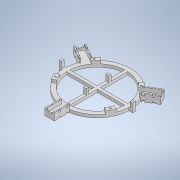
# Autodesk Inventor part: bottom2
Saved by Autodesk Inventor 2020.2 (Build 242310000, 310)
## iProperties
Created: 2020-03-22
Part Number: bottom2
Material: Generic
Document SubType Name: Modeling
Designer: Tarsoly
Density: 1 g/cm^3
Appearance: Default
Author: Tarsoly
Autodesk Inventor part; units mm, degrees
ref_plane "YZ Plane" through (0, 0, 0) normal (1, 0, 0) x (0, 1, 0)
sketch "Sketch1" plane through (0, 0, 0) normal (0, 1, 0) x (-1, 0, 0)
  circle A0 centre (0, 0) radius 57
  circle A1 centre (0, 0) radius 50
  line L0 (0, -84.8) -> (0, 109.8) construction
  line L1 (105.0197, 0) -> (-105.0197, 0) construction
  line L2 (8, 82) -> (-8, 82)
  line L3 (-8, 82) -> (-8, 50)
  line L4 (-8, 50) -> (8, 50)
  line L5 (8, 50) -> (8, 82)
  line L6 (0, 82) -> (0, 50) construction
  circle A2 centre (0, 0) radius 53.5 construction
  circle A3 centre (40.4629, -35) radius 1.5
  circle A4 centre (-40.4629, -35) radius 1.5
  circle A5 centre (-47.2996, 25) radius 1.5
  circle A6 centre (47.2996, 25) radius 1.5
  line L7 (-75.0141, -34.0718) -> (-67.0141, -47.9282)
  line L8 (-39.3013, -31.9282) -> (-47.3013, -18.0718)
  line L9 (-67.0141, -47.9282) -> (-39.3013, -31.9282)
  line L10 (-71.0141, -41) -> (-43.3013, -25) construction
  line L11 (-47.3013, -18.0718) -> (-75.0141, -34.0718)
  line L12 (67.0141, -47.9282) -> (75.0141, -34.0718)
  line L13 (47.3013, -18.0718) -> (39.3013, -31.9282)
  line L14 (75.0141, -34.0718) -> (47.3013, -18.0718)
  line L15 (71.0141, -41) -> (43.3013, -25) construction
  line L16 (39.3013, -31.9282) -> (67.0141, -47.9282)
  point P0 (-8, 56.4358)
  point P1 (8, 56.4358)
  point P2 (-44.8748, -35.1461)
  point P3 (-52.8748, -21.2897)
  point P4 (52.8748, -21.2897)
  point P5 (44.8748, -35.1461)
  dimension "d0" = 114
  dimension "d1" = 100
  dimension "d10" = 16
  dimension "d61" = 107
  dimension "d62" = 3
  dimension "d63" = 3
  dimension "d64" = 3
  dimension "d65" = 3
  dimension "d66" = 35
  dimension "d67" = 35
  dimension "d68" = 25
  dimension "d69" = 25
  dimension "d71" = 32
  dimension "d92" = 360
  constraints: 30 end point, 7 centre point, 4 point on circle, 3 coincident, 2 midpoint, 2 parallel, 1 collinear, 1 horizontal, 1 perpendicular, 1 tangent, 34 other
  measures "d0" diameter of A0
  measures "d1" diameter of A1
  measures "d10" distance of L4.end L3.end
  measures "d61" diameter of A2
  measures "d62" diameter of A3
  measures "d63" diameter of A4
  measures "d64" diameter of A5
  measures "d65" diameter of A6
  measures "d66" distance from line of L1 A3.centre
  measures "d67" distance from line of L1 A4.centre
  measures "d68" distance from line of L1 A5.centre
  measures "d69" distance from line of L1 A6.centre
  measures "d71" distance between parallel lines of L4 L2
extrude "Extrusion1" add sketch "Sketch1" along normal blind 5 contours A0 L14 L13 A1 L4 L5 | L5 L4 L3 A0 | A0 L3 L2 L5 | L14 L12 L16 A0 | A0 L16 L13 L14 | L3 L4 A1 L8 L11 A0 | A0 L9 L8 A1 L13 L16 | L11 L8 L9 A0 | A0 L9 L7 L11
sketch "Sketch8" plane through (0, 0, 0) normal (0, -1, 0) x (1, 0, 0)
  line L0 (59, 17) -> (-59, 17) construction
  line L1 (-59, 17) -> (-59, -17) construction
  line L2 (-59, -17) -> (59, -17) construction
  line L3 (59, -17) -> (59, 17) construction
  line L4 (59, 17) -> (-59, -17) construction
  line L5 (-59, 17) -> (59, -17) construction
  line L6 (63.2, 2.5) -> (-63.2, 2.5)
  line L7 (-63.2, 2.5) -> (-63.2, -2.5)
  line L8 (-63.2, -2.5) -> (63.2, -2.5)
  line L9 (63.2, -2.5) -> (63.2, 2.5)
  line L10 (63.2, 2.5) -> (-63.2, -2.5) construction
  line L11 (-63.2, 2.5) -> (63.2, -2.5) construction
  line L12 (-2.5, 50) -> (2.5, 50)
  line L13 (2.5, 50) -> (2.5, -50)
  line L14 (2.5, -50) -> (-2.5, -50)
  line L15 (-2.5, -50) -> (-2.5, 50)
  line L16 (-2.5, 50) -> (2.5, -50) construction
  line L17 (2.5, 50) -> (-2.5, -50) construction
  circle A0 centre (0, 0) radius 50 projected
  point P0 (2.5, 2.5)
  point P1 (-2.5, 2.5)
  point P2 (-2.5, -2.5)
  point P3 (2.5, -2.5)
  dimension "d98" = 118
  dimension "d99" = 34
  dimension "d100" = 5
  dimension "d101" = 4.2
  dimension "d102" = 5
  constraints: 36 end point, 6 midpoint, 6 parallel, 3 horizontal, 3 perpendicular, 1 tangent
  measures "d98" distance of L2.end L1.end
  measures "d99" distance of L1.end L0.end
  measures "d100" distance of L7.end L6.end
  measures "d101" distance between parallel lines of L1 L7
  measures "d102" distance between parallel lines of L15 L13
extrude "Extrusion7" add sketch "Sketch8" against normal blind 5 contours L9 L8 A0 L6 | A0 L8 L13 L6 | L13 L8 L15 L6 | L6 L15 A0 L13 | A0 L12 L13 | L15 L8 A0 L6 | L13 A0 L15 L8 | A0 L15 L12 | L13 L14 A0 | A0 L8 L7 L6 | L14 L15 A0
sketch "Sketch9" plane through (0, 5, 0) normal (0, 1, 0) x (1, 0, 0)
  line L0 (-59, 17) -> (59, 17) construction
  line L1 (59, 17) -> (59, -17) construction
  line L2 (59, -17) -> (-59, -17) construction
  line L3 (-59, -17) -> (-59, 17) construction
  line L4 (-59, 17) -> (59, -17) construction
  line L5 (59, 17) -> (-59, -17) construction
  line L6 (-63.2, -2.5) -> (-63.2, 2.5) projected
  line L7 (-63.2, -2.5) -> (-56.9451, -2.5) construction
  line L8 (-63.2, 2.5) -> (-59.2, 2.5)
  line L9 (-59.2, 2.5) -> (-59.2, -2.5)
  line L10 (-59.2, -2.5) -> (-63.2, -2.5)
  line L11 (-63.2, -2.5) -> (-63.2, 2.5)
  line L12 (0, 84.8) -> (0, -109.8) construction
  line L13 (-105.0197, 0) -> (105.0197, 0) construction
  line L14 (63.2, -2.5) -> (63.2, 2.5)
  line L15 (63.2, 2.5) -> (59.2, 2.5)
  line L16 (59.2, 2.5) -> (59.2, -2.5)
  line L17 (59.2, -2.5) -> (63.2, -2.5)
  line L18 (63.2, -2.5) -> (63.2, 2.5)
  line L19 (-2.5, -49.9375) -> (-2.5, -2.5) construction
  line L20 (2.5, -2.5) -> (2.5, -49.9375) construction
  line L21 (-2.5, -21.2) -> (2.5, -21.2)
  line L22 (2.5, -21.2) -> (2.5, -17.2)
  line L23 (2.5, -17.2) -> (-2.5, -17.2)
  line L24 (-2.5, -17.2) -> (-2.5, -21.2)
  line L25 (-2.5, 21.2) -> (2.5, 21.2)
  line L26 (2.5, 21.2) -> (2.5, 17.2)
  line L27 (2.5, 17.2) -> (-2.5, 17.2)
  line L28 (-2.5, 17.2) -> (-2.5, 21.2)
  point P0 (0, 0)
  dimension "d105" = 118
  dimension "d106" = 34
  dimension "d108" = 4
  dimension "d109" = 0.2
  dimension "d112" = 0.2
  constraints: 46 end point, 9 symmetric about line, 6 parallel, 3 horizontal, 3 perpendicular, 3 point on line, 2 midpoint
  measures "d105" distance of L1.end L2.end
  measures "d106" distance of L0.end L1.end
  measures "d108" distance of L22.end L21.end
  measures "d109" distance between parallel lines of L2 L23
  measures "d112" distance between parallel lines of L3 L9
extrude "Extrusion8" add sketch "Sketch9" along normal blind 10
sketch "Sketch6" plane through (0, 5, 0) normal (0, 1, 0) x (1, 0, 0)
  line L0 (-8, -82) -> (8, -82) projected
  line L1 (8, -82) -> (8, -56.4358) projected
  line L2 (-8, -82) -> (8, -82)
  line L3 (8, -82) -> (8, -55)
  line L4 (8, -55) -> (-8, -55)
  line L5 (-8, -55) -> (-8, -82)
  line L6 (-6, -80) -> (6, -80)
  line L7 (6, -80) -> (6, -57)
  line L8 (6, -57) -> (-6, -57)
  line L9 (-6, -57) -> (-6, -80)
  line L10 (-6, -57) -> (-6, -55)
  line L11 (6, -57) -> (6, -55)
  point P0 (0, 0)
  dimension "d46" = 27
  dimension "d47" = 2
  constraints: 20 end point, 4 parallel, 4 point on line, 3 perpendicular, 1 horizontal, 3 other
  measures "d46" distance between parallel lines of L0 L4
  measures "d47" distance between parallel lines of L5 L9
extrude "Extrusion5" add sketch "Sketch6" along normal blind 7 contours L5 L4 L10 L9 L6 L7 L11 L3 L1 L0
sketch "Sketch7" plane through (-8, 0, 82) normal (0, 0, 1) x (1, 0, 0)
  line L0 (2, 5) -> (2, 5) projected
  circle A0 centre (8, 10) radius 2.5
  line L1 (3.5, 10) -> (8, 10) construction
  line L2 (8, 10) -> (12.5, 10) construction
  circle A1 centre (3.5, 10) radius 1
  circle A2 centre (12.5, 10) radius 1
  line L3 (3.5, 11) -> (5.7087, 11)
  line L4 (3.5, 9) -> (5.7087, 9)
  line L5 (10.2913, 11) -> (12.5, 11)
  line L6 (10.2913, 9) -> (12.5, 9)
  line L7 (0, 12) -> (16, 12) projected
  line L8 (2.5, 12) -> (2.5, 10)
  line L9 (13.5, 12) -> (13.5, 10)
  line L10 (0, 0) -> (0, 5) construction
  line L11 (-44.8748, 5) -> (16, 5) construction
  line L12 (0, 5) -> (16, 5) construction
  line L13 (52.8748, 5) -> (-36.8748, 5) projected
  line L14 (8, 5) -> (8, 10)
  point P0 (9.5, 12)
  point P1 (6.5, 12)
  point P2 (60.8748, 5)
  dimension "d51" = 5
  dimension "d53" = 9
  dimension "d54" = 2
  dimension "d55" = 2
  dimension "d94" = 5
  constraints: 20 end point, 10 point on circle, 6 tangent, 5 horizontal, 3 centre point, 3 point on line, 2 coincident, 2 parallel, 1 collinear, 1 midpoint, 1 perpendicular, 1 vertical, 1 other
  measures "d51" diameter of A0
  measures "d53" distance of L2.end L1.start
  measures "d54" diameter of A1
  measures "d55" diameter of A2
  measures "d94" distance of L14.start L1.end
extrude "Extrusion6" cut sketch "Sketch7" against normal up to surface (2 mm away)
ref_plane "Work Plane1" through (6, 5, 73) normal (0, 0, -1) x (-1, 0, 0)
ref_plane "Work Plane2" through (6, 5, 58) normal (0, 0, -1) x (-1, 0, 0)
sketch "Sketch14" plane through (6, 5, 73) normal (0, 0, -1) x (-1, 0, 0)
  line L0 (0, 0) -> (-2, 0) projected
  line L1 (0, 0) -> (0, 7) projected
  line L2 (-2, 7) -> (0, 7) projected
  line L3 (-2, 0) -> (-2, 7) projected
  line L4 (0, 7) -> (-2, 4)
  line L5 (-2, 0) -> (-2, 7) projected
  line L6 (-2, 7) -> (0, 7) projected
  line L7 (-2, 7) -> (0, 7)
  line L8 (6, -8) -> (6, 13) construction
  line L9 (14, 7) -> (12, 7)
  line L10 (14, 0) -> (14, 7)
  line L11 (12, 7) -> (14, 4)
  line L12 (50.8748, -5) -> (-38.8748, -5) projected
  line L13 (-2, -5) -> (-2, -3)
  line L14 (-2, -3) -> (0, -5)
  line L15 (0, -5) -> (-2, -5)
  line L16 (-2, -5) -> (-2, 7) projected
  line L17 (14, -5) -> (14, -3)
  line L18 (14, -3) -> (12, -5)
  line L19 (12, -5) -> (14, -5)
  point P0 (6, -5)
  point P1 (0, -5)
  dimension "d138" = 3
  dimension "d143" = 2
  dimension "d144" = 45
  constraints: 22 end point, 7 symmetric about line, 3 point on line, 2 perpendicular, 1 horizontal
  measures "d138" distance from line of L4.end L2
  measures "d143" distance of L13.start L13.end
  measures "d144" angle of L13 L14
extrude "Extrusion12" cut sketch "Sketch14" along normal mid plane 3.6 contours L4 L3 L2 | L10 L11 L9 | L12 L18 L17 | L12 L13 L14
sketch "Sketch15" plane through (6, 5, 58) normal (0, 0, -1) x (-1, 0, 0)
  line L0 (0, 7) -> (-2, 4) projected
  line L1 (-2, 7) -> (0, 7) projected
  line L2 (-2, 4) -> (-2, 7) projected
  line L3 (12, 7) -> (14, 4) projected
  line L4 (14, 7) -> (12, 7) projected
  line L5 (14, 4) -> (14, 7) projected
  line L6 (-2, -3) -> (-2, -5) projected
  line L7 (0, -5) -> (-2, -3) projected
  line L8 (-2, -5) -> (0, -5) projected
  line L9 (12, -5) -> (14, -5) projected
  line L10 (14, -3) -> (12, -5) projected
  line L11 (14, -5) -> (14, -3) projected
  point P0 (6, -5)
extrude "Extrusion13" cut sketch "Sketch15" against normal blind 3.6
pattern_circular "Circular Pattern3" count 3 over 360 about axis through (0, -10, 0) along (0, 1, 0) of "Extrusion5", "Extrusion6", "Extrusion12", "Extrusion13"
sketch "Sketch10" plane through (0, 5, 0) normal (0, 1, 0) x (1, 0, 0)
  line L0 (-44.8748, 35.1461) -> (-43.6314, 34.4282) projected
  line L1 (-43.6314, 34.4282) -> (-44.6314, 32.6962) projected
  line L2 (-44.6314, 32.6962) -> (-66.282, 45.1962) projected
  line L3 (-66.282, 45.1962) -> (-72.282, 34.8038) projected
  line L4 (-72.282, 34.8038) -> (-50.6314, 22.3038) projected
  line L5 (-50.6314, 22.3038) -> (-51.6314, 20.5718) projected
  line L6 (-51.6314, 20.5718) -> (-52.8748, 21.2897) projected
  arc A0 (-52.8748, 21.2897) -> (-56.9451, 2.5) centre (0, 0) ccw projected
  line L7 (-56.9451, 2.5) -> (-59.2, 2.5) projected
  line L8 (-59.2, 2.5) -> (-59.2, -2.5) projected
  line L9 (-59.2, -2.5) -> (-56.9451, -2.5) projected
  arc A1 (-56.9451, -2.5) -> (-8, -56.4358) centre (0, 0) ccw projected
  line L10 (-8, -56.4358) -> (-8, -55) projected
  line L11 (-8, -55) -> (-6, -55) projected
  line L12 (-6, -55) -> (-6, -80) projected
  line L13 (-6, -80) -> (6, -80) projected
  line L14 (6, -80) -> (6, -55) projected
  line L15 (6, -55) -> (8, -55) projected
  line L16 (8, -55) -> (8, -56.4358) projected
  arc A2 (8, -56.4358) -> (56.9451, -2.5) centre (0, 0) ccw projected
  line L17 (56.9451, -2.5) -> (59.2, -2.5) projected
  line L18 (59.2, -2.5) -> (59.2, 2.5) projected
  line L19 (59.2, 2.5) -> (56.9451, 2.5) projected
  arc A3 (56.9451, 2.5) -> (52.8748, 21.2897) centre (0, 0) ccw projected
  line L20 (52.8748, 21.2897) -> (51.6314, 20.5718) projected
  line L21 (51.6314, 20.5718) -> (50.6314, 22.3038) projected
  line L22 (50.6314, 22.3038) -> (72.282, 34.8038) projected
  line L23 (72.282, 34.8038) -> (66.282, 45.1962) projected
  line L24 (66.282, 45.1962) -> (44.6314, 32.6962) projected
  line L25 (44.6314, 32.6962) -> (43.6314, 34.4282) projected
  line L26 (43.6314, 34.4282) -> (44.8748, 35.1461) projected
  arc A4 (44.8748, 35.1461) -> (-44.8748, 35.1461) centre (0, 0) ccw projected
  line L27 (2.5, 17.2) -> (-2.5, 17.2) projected
  line L28 (-2.5, 17.2) -> (-2.5, 2.5) projected
  line L29 (-2.5, 2.5) -> (-49.9375, 2.5) projected
  arc A5 (-2.5, 49.9375) -> (-49.9375, 2.5) centre (0, 0) ccw projected
  line L30 (-2.5, 49.9375) -> (-2.5, 21.2) projected
  line L31 (-2.5, 21.2) -> (2.5, 21.2) projected
  line L32 (2.5, 21.2) -> (2.5, 49.9375) projected
  arc A6 (49.9375, 2.5) -> (2.5, 49.9375) centre (0, 0) ccw projected
  line L33 (49.9375, 2.5) -> (2.5, 2.5) projected
  line L34 (2.5, 2.5) -> (2.5, 17.2) projected
  line L35 (2.5, -21.2) -> (-2.5, -21.2) projected
  line L36 (-2.5, -21.2) -> (-2.5, -49.9375) projected
  arc A7 (-49.9375, -2.5) -> (-2.5, -49.9375) centre (0, 0) ccw projected
  line L37 (-49.9375, -2.5) -> (-2.5, -2.5) projected
  line L38 (-2.5, -2.5) -> (-2.5, -17.2) projected
  line L39 (-2.5, -17.2) -> (2.5, -17.2) projected
  line L40 (2.5, -17.2) -> (2.5, -2.5) projected
  line L41 (2.5, -2.5) -> (49.9375, -2.5) projected
  arc A8 (2.5, -49.9375) -> (49.9375, -2.5) centre (0, 0) ccw projected
  line L42 (2.5, -49.9375) -> (2.5, -21.2) projected
  circle A9 centre (47.2996, -25) radius 1.5 projected
  circle A10 centre (-47.2996, -25) radius 1.5 projected
  circle A11 centre (-40.4629, 35) radius 1.5 projected
  circle A12 centre (40.4629, 35) radius 1.5 projected
  arc A13 (-49.9375, -2.5) -> (-2.5, -49.9375) centre (0, 0) ccw projected
  line L43 (-46.8675, -17.4195) -> (-53.1026, -20.7151)
  arc A14 (-56.9451, -2.5) -> (-8, -56.4358) centre (0, 0) ccw projected
  line L44 (-40.7927, -28.9129) -> (-47.0278, -32.2084)
  line L45 (0, 0) -> (-47.2996, -25) construction
  line L46 (0, 0) -> (40.4629, 35) construction
  line L47 (0, 0) -> (47.2996, -25) construction
  line L48 (0, 0) -> (-40.4629, 35) construction
  line L49 (-43.6314, 34.4282) -> (-44.6314, 32.6962) projected
  line L50 (-44.6314, 32.6962) -> (-39.9884, 30.0155)
  arc A15 (-2.5, 49.9375) -> (-49.9375, 2.5) centre (0, 0) ccw projected
  line L51 (-32.095, 38.3394) -> (-37.4497, 42.9712)
  arc A16 (44.8748, 35.1461) -> (-44.8748, 35.1461) centre (0, 0) ccw projected
  line L52 (44.6314, 32.6962) -> (39.9884, 30.0155)
  arc A17 (49.9375, 2.5) -> (2.5, 49.9375) centre (0, 0) ccw projected
  line L53 (44.6314, 32.6962) -> (66.282, 45.1962) projected
  line L54 (32.095, 38.3394) -> (37.4497, 42.9712)
  arc A18 (2.5, -49.9375) -> (49.9375, -2.5) centre (0, 0) ccw projected
  line L55 (40.7927, -28.9129) -> (47.0278, -32.2084)
  line L56 (46.8675, -17.4195) -> (53.1026, -20.7151)
  dimension "d113" = 13
  dimension "d114" = 8
  dimension "d115" = 8
  dimension "d116" = 13
  constraints: 24 end point, 14 point on circle, 6 parallel, 1 collinear, 1 perpendicular, 2 other
  measures "d113" distance between parallel lines of L44 L43
  measures "d114" distance between parallel lines of L51 L48
  measures "d115" distance between parallel lines of L54 L46
  measures "d116" distance between parallel lines of L56 L55
extrude "Extrusion9" add sketch "Sketch10" along normal blind 5 contours A4 L51 A5 L50 L1 L0 | A4 L26 L25 L52 A6 L54 | L43 A7 L44 A1 | A2 L55 A8 L56
sketch "Sketch11" plane through (0, 0, 0) normal (0, -1, 0) x (1, 0, 0)
  arc A0 (-49.9375, -2.5) -> (-2.5, -49.9375) centre (0, 0) ccw projected
  line L0 (-49.9375, -2.5) -> (-2.5, -2.5) projected
  line L1 (-2.5, -2.5) -> (-2.5, -49.9375) projected
  line L2 (2.5, -49.9375) -> (2.5, -2.5) projected
  line L3 (2.5, -2.5) -> (49.9375, -2.5) projected
  arc A1 (2.5, -49.9375) -> (49.9375, -2.5) centre (0, 0) ccw projected
  line L4 (49.9375, 2.5) -> (2.5, 2.5) projected
  line L5 (2.5, 2.5) -> (2.5, 49.9375) projected
  arc A2 (49.9375, 2.5) -> (2.5, 49.9375) centre (0, 0) ccw projected
  line L6 (-2.5, 49.9375) -> (-2.5, 2.5) projected
  line L7 (-2.5, 2.5) -> (-49.9375, 2.5) projected
  arc A3 (-2.5, 49.9375) -> (-49.9375, 2.5) centre (0, 0) ccw projected
  circle A4 centre (47.2996, 25) radius 1.5 projected
  circle A5 centre (-47.2996, 25) radius 1.5 projected
  arc A6 (56.9451, 2.5) -> (8, 56.4358) centre (0, 0) ccw projected
  line L8 (8, 82) -> (8, 74.8) projected
  line L9 (-8, 82) -> (8, 82) projected
  line L10 (-8, 56.4358) -> (-8, 58) projected
  arc A7 (-8, 56.4358) -> (-56.9451, 2.5) centre (0, 0) ccw projected
  line L11 (-56.9451, 2.5) -> (-63.2, 2.5) projected
  line L12 (-63.2, 2.5) -> (-63.2, -2.5) projected
  line L13 (-63.2, -2.5) -> (-56.9451, -2.5) projected
  arc A8 (-56.9451, -2.5) -> (-52.8748, -21.2897) centre (0, 0) ccw projected
  line L14 (-75.0141, -34.0718) -> (-68.7787, -30.4718) projected
  line L15 (-67.0141, -47.9282) -> (-75.0141, -34.0718) projected
  line L16 (-44.8748, -35.1461) -> (-46.2295, -35.9282) projected
  arc A9 (-44.8748, -35.1461) -> (44.8748, -35.1461) centre (0, 0) ccw projected
  line L17 (67.0141, -47.9282) -> (60.7787, -44.3282) projected
  line L18 (75.0141, -34.0718) -> (67.0141, -47.9282) projected
  line L19 (52.8748, -21.2897) -> (54.2295, -22.0718) projected
  arc A10 (52.8748, -21.2897) -> (56.9451, -2.5) centre (0, 0) ccw projected
  line L20 (56.9451, -2.5) -> (63.2, -2.5) projected
  line L21 (63.2, -2.5) -> (63.2, 2.5) projected
  line L22 (63.2, 2.5) -> (56.9451, 2.5) projected
  circle A11 centre (40.4629, -35) radius 1.5 projected
  circle A12 centre (-40.4629, -35) radius 1.5 projected
  line L23 (6, 61.6) -> (8, 61.6) projected
  line L24 (8, 71.2) -> (8, 61.6) projected
  line L25 (8, 71.2) -> (6, 71.2) projected
  line L26 (6, 71.2) -> (6, 74.8) projected
  line L27 (6, 74.8) -> (8, 74.8) projected
  line L28 (-8, 74.8) -> (-8, 82) projected
  line L29 (-8, 74.8) -> (-6, 74.8) projected
  line L30 (-6, 74.8) -> (-6, 71.2) projected
  line L31 (-6, 71.2) -> (-8, 71.2) projected
  line L32 (-8, 61.6) -> (-8, 71.2) projected
  line L33 (-8, 61.6) -> (-6, 61.6) projected
  line L34 (-6, 61.6) -> (-6, 58) projected
  line L35 (-6, 58) -> (-8, 58) projected
  line L36 (8, 58) -> (8, 56.4358) projected
  line L37 (8, 58) -> (6, 58) projected
  line L38 (6, 58) -> (6, 61.6) projected
  line L39 (-58.661, -40.7962) -> (-57.661, -42.5282) projected
  line L40 (-49.3472, -37.7282) -> (-57.661, -42.5282) projected
  line L41 (-49.3472, -37.7282) -> (-50.3472, -35.9962) projected
  line L42 (-50.3472, -35.9962) -> (-47.2295, -34.1962) projected
  line L43 (-47.2295, -34.1962) -> (-46.2295, -35.9282) projected
  line L44 (46.2295, -35.9282) -> (44.8748, -35.1461) projected
  line L45 (46.2295, -35.9282) -> (47.2295, -34.1962) projected
  line L46 (47.2295, -34.1962) -> (50.3472, -35.9962) projected
  line L47 (50.3472, -35.9962) -> (49.3472, -37.7282) projected
  line L48 (57.661, -42.5282) -> (49.3472, -37.7282) projected
  line L49 (57.661, -42.5282) -> (58.661, -40.7962) projected
  line L50 (58.661, -40.7962) -> (61.7787, -42.5962) projected
  line L51 (61.7787, -42.5962) -> (60.7787, -44.3282) projected
  line L52 (68.7787, -30.4718) -> (75.0141, -34.0718) projected
  line L53 (68.7787, -30.4718) -> (67.7787, -32.2038) projected
  line L54 (67.7787, -32.2038) -> (64.661, -30.4038) projected
  line L55 (64.661, -30.4038) -> (65.661, -28.6718) projected
  line L56 (57.3472, -23.8718) -> (65.661, -28.6718) projected
  line L57 (57.3472, -23.8718) -> (56.3472, -25.6038) projected
  line L58 (56.3472, -25.6038) -> (53.2295, -23.8038) projected
  line L59 (53.2295, -23.8038) -> (54.2295, -22.0718) projected
  line L60 (-54.2295, -22.0718) -> (-52.8748, -21.2897) projected
  line L61 (-54.2295, -22.0718) -> (-53.2295, -23.8038) projected
  line L62 (-53.2295, -23.8038) -> (-56.3472, -25.6038) projected
  line L63 (-56.3472, -25.6038) -> (-57.3472, -23.8718) projected
  line L64 (-65.661, -28.6718) -> (-57.3472, -23.8718) projected
  line L65 (-65.661, -28.6718) -> (-64.661, -30.4038) projected
  line L66 (-64.661, -30.4038) -> (-67.7787, -32.2038) projected
  line L67 (-67.7787, -32.2038) -> (-68.7787, -30.4718) projected
  line L68 (-60.7787, -44.3282) -> (-67.0141, -47.9282) projected
  line L69 (-60.7787, -44.3282) -> (-61.7787, -42.5962) projected
  line L70 (-61.7787, -42.5962) -> (-58.661, -40.7962) projected
hole "Hole1" at (-47.2996, 0, 25) at (47.2996, 0, 25) at (40.4629, 0, -35) at (-40.4629, 0, -35) direction (0, 1, 0) diameter 6 depth 5 tip angle 118 clearance for "Hex Head Cap Screw ISO 24017" size "M6" standard "ISO"
equation "\"d61\" = 0.5 * d1 + 0.5 * d0"
body "Solid1"
